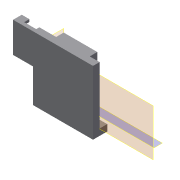
# Autodesk Inventor part: 10_Minispim_Base
Saved by Autodesk Inventor 2019 (Build 230136000, 136)
## iProperties
Created: 2019-08-27
Part Number: 10_Minispim_Base
Material: Generic
Document SubType Name: Modeling
Designer: diederichbenedict
Density: 1 g/cm^3
Appearance: Default
Author: diederichbenedict
Autodesk Inventor part; units mm, degrees
ref_plane "YZ Plane" through (0, 0, 0) normal (1, 0, 0) x (0, 1, 0)
ref_plane "XZ Plane" through (0, 0, 0) normal (0, 1, 0) x (-1, 0, 0)
ref_plane "XY Plane" through (0, 0, 0) normal (0, 0, 1) x (1, 0, 0)
ref_plane "Work Plane1" through (0, 0, 0) normal (0, 0, 1) x (1, 0, 0)
sketch "Sketch1" plane through (0, 0, 0) normal (0, 0, 1) x (1, 0, 0)
  line L0 (73, -36.65) -> (-73, -36.65) construction
  line L1 (73, 36.65) -> (73, -36.65) construction
  line L2 (-73, 36.65) -> (73, 36.65) construction
  line L3 (-73, -36.65) -> (-73, 36.65) construction
  line L4 (-66.8632, 12.8749) -> (-66.8632, 14.232) construction
  line L5 (-66.8632, 14.232) -> (-61.4969, 10.9795) construction
  line L6 (-61.4969, 10.9795) -> (-57.2382, 10.9795) construction
  line L7 (-57.2382, 10.9795) -> (-57.2382, 9.7003) construction
  line L8 (-57.2382, 9.7003) -> (-61.3643, 9.7003) construction
  line L9 (-61.3643, 9.7003) -> (-66.8632, 6.4478) construction
  line L10 (-66.8632, 6.4478) -> (-66.8632, 7.8674) construction
  line L11 (-66.8632, 7.8674) -> (-62.6279, 10.3477) construction
  line L12 (-62.6279, 10.3477) -> (-66.8632, 12.8749) construction
  spline S0 degree 2 poles (-57.9402, -12.888) (-57.519, -13.3482) (-57.0666, -14.5182) (-57.0666, -15.3995) knots 0 0 0 1 2 2 2 construction
  spline S1 degree 2 poles (-57.0666, -15.3995) (-57.0666, -16.4447) (-57.5034, -17.9111) (-57.8154, -18.5585) knots 0 0 0 1 2 2 2 construction
  line L13 (-57.8154, -18.5585) -> (-59.4221, -18.5585) construction
  line L14 (-59.4221, -18.5585) -> (-59.4221, -18.4649) construction
  spline S2 degree 2 poles (-59.4221, -18.4649) (-58.8294, -17.8331) (-58.1742, -16.2341) (-58.1742, -15.4931) knots 0 0 0 1 2 2 2 construction
  spline S3 degree 2 poles (-58.1742, -15.4931) (-58.1742, -14.4324) (-59.0555, -13.3482) (-59.7809, -13.3482) knots 0 0 0 1 2 2 2 construction
  spline S4 degree 2 poles (-59.7809, -13.3482) (-60.3581, -13.3482) (-61.0757, -13.9176) (-61.2551, -14.5338) knots 0 0 0 1 2 2 2 construction
  spline S5 degree 2 poles (-61.2551, -14.5338) (-61.3799, -14.9784) (-61.5515, -15.7193) (-61.6919, -16.2731) knots 0 0 0 1 2 2 2 construction
  spline S6 degree 2 poles (-61.6919, -16.2731) (-61.8245, -16.7723) (-62.2223, -17.5601) (-62.5421, -17.8643) knots 0 0 0 1 2 2 2 construction
  spline S7 degree 2 poles (-62.5421, -17.8643) (-62.8619, -18.1607) (-63.7199, -18.4883) (-64.2814, -18.4883) knots 0 0 0 1 2 2 2 construction
  spline S8 degree 2 poles (-64.2814, -18.4883) (-65.4514, -18.4883) (-67.0348, -16.6631) (-67.0348, -15.2514) knots 0 0 0 1 2 2 2 construction
  spline S9 degree 2 poles (-67.0348, -15.2514) (-67.0348, -14.4402) (-66.715, -13.005) (-66.4108, -12.3888) knots 0 0 0 1 2 2 2 construction
  line L15 (-66.4108, -12.3888) -> (-64.882, -12.3888) construction
  line L16 (-64.882, -12.3888) -> (-64.882, -12.4824) construction
  spline S10 degree 2 poles (-64.882, -12.4824) (-65.3032, -12.9426) (-65.9272, -14.3778) (-65.9272, -15.1656) knots 0 0 0 1 2 2 2 construction
  spline S11 degree 2 poles (-65.9272, -15.1656) (-65.9272, -16.0547) (-65.0926, -17.1545) (-64.414, -17.1545) knots 0 0 0 1 2 2 2 construction
  spline S12 degree 2 poles (-64.414, -17.1545) (-63.8057, -17.1545) (-63.0803, -16.5071) (-62.9165, -15.8987) knots 0 0 0 1 2 2 2 construction
  spline S13 degree 2 poles (-62.9165, -15.8987) (-62.8073, -15.4931) (-62.5265, -14.3154) (-62.4095, -13.9254) knots 0 0 0 1 2 2 2 construction
  spline S14 degree 2 poles (-62.4095, -13.9254) (-62.1053, -12.9348) (-60.8807, -12.0144) (-59.9837, -12.0144) knots 0 0 0 1 2 2 2 construction
  spline S15 degree 2 poles (-59.9837, -12.0144) (-59.4143, -12.0144) (-58.3224, -12.4746) (-57.9402, -12.888) knots 0 0 0 1 2 2 2 construction
  spline S16 degree 2 poles (-67.066, -7.0069) (-67.066, -6.0241) (-66.3796, -4.4486) (-65.7634, -3.9026) knots 0 0 0 1 2 2 2 construction
  spline S17 degree 2 poles (-65.7634, -3.9026) (-65.1238, -3.3566) (-63.2519, -2.7482) (-62.0507, -2.7482) knots 0 0 0 1 2 2 2 construction
  spline S18 degree 2 poles (-62.0507, -2.7482) (-60.8807, -2.7482) (-58.9854, -3.341) (-58.3458, -3.9026) knots 0 0 0 1 2 2 2 construction
  spline S19 degree 2 poles (-58.3458, -3.9026) (-57.675, -4.4954) (-57.0354, -6.0631) (-57.0354, -7.0069) knots 0 0 0 1 2 2 2 construction
  spline S20 degree 2 poles (-57.0354, -7.0069) (-57.0354, -7.9819) (-57.6984, -9.5419) (-58.3458, -10.1113) knots 0 0 0 1 2 2 2 construction
  spline S21 degree 2 poles (-58.3458, -10.1113) (-58.9854, -10.665) (-60.8651, -11.2578) (-62.0507, -11.2578) knots 0 0 0 1 2 2 2 construction
  spline S22 degree 2 poles (-62.0507, -11.2578) (-63.2597, -11.2578) (-65.1004, -10.6572) (-65.7634, -10.1035) knots 0 0 0 1 2 2 2 construction
  spline S23 degree 2 poles (-65.7634, -10.1035) (-66.403, -9.5419) (-67.066, -7.9741) (-67.066, -7.0069) knots 0 0 0 1 2 2 2 construction
  line L17 (-66.8632, 5.543) -> (-57.2382, 5.543) construction
  line L18 (-57.2382, 5.543) -> (-57.2382, 4.1078) construction
  line L19 (-57.2382, 4.1078) -> (-65.5372, -0.1509) construction
  line L20 (-65.5372, -0.1509) -> (-57.2382, -0.1509) construction
  line L21 (-57.2382, -0.1509) -> (-57.2382, -1.3442) construction
  line L22 (-57.2382, -1.3442) -> (-66.8632, -1.3442) construction
  line L23 (-66.8632, -1.3442) -> (-66.8632, 0.4731) construction
  line L24 (-66.8632, 0.4731) -> (-59.2427, 4.3496) construction
  line L25 (-59.2427, 4.3496) -> (-66.8632, 4.3496) construction
  line L26 (-66.8632, 4.3496) -> (-66.8632, 5.543) construction
  line L27 (-75, -25.3081) -> (-75, -38.65) construction
  line L28 (-75, -38.65) -> (75, -38.65) construction
  line L29 (-75, 38.65) -> (-75, -16.9919) construction
  line L30 (75, 38.65) -> (-75, 38.65) construction
  line L31 (-151.75, -50.65) -> (-11.75, -50.65)
  line L32 (-11.75, -50.65) -> (-11.75, 59.35)
  line L33 (-11.75, 59.35) -> (-151.75, 59.35)
  line L34 (-151.75, 59.35) -> (-151.75, -50.65)
  line L35 (-146.75, 47.05) -> (-146.75, 14.683) construction
  line L36 (-11.75, -50.65) -> (-75, -50.65)
  line L37 (-75, -50.65) -> (-75, 59.35)
  line L38 (-75, 59.35) -> (-11.75, 59.35)
  line L39 (-11.75, 59.35) -> (-11.75, -50.65)
  point P0 (0, 0)
  dimension "d0" = 140
  dimension "d1" = 110
  dimension "d2" = 12
  dimension "d3" = 5
  constraints: 16 end point, 4 parallel, 2 horizontal, 2 perpendicular, 1 point on line
  measures "d0" distance of L33.end L32.end
  measures "d1" distance of L32.end L31.end
  measures "d2" distance between parallel lines of L31 L28
  measures "d3" distance between parallel lines of L35 L34
ref_plane "Work Plane2" through (-137.8164, 12.7477, 6.4) normal (0, 0, 1) x (1, 0, 0)
extrude "Extrusion1" add sketch "Sketch1" along normal up to surface (6.4 mm away) contours L37 L33 L32 L31
sketch "Sketch2" plane through (0, 0, 0) normal (0, 0, -1) x (-1, 0, 0)
  line L0 (11.75, -50.65) -> (11.75, 59.35) projected
  line L1 (75, -50.65) -> (11.75, -50.65) projected
  line L2 (75, 59.35) -> (75, -50.65) projected
  line L3 (11.75, 59.35) -> (75, 59.35) projected
  line L4 (75, 38.65) -> (-75, 38.65) projected
  line L5 (75, -38.65) -> (-75, -38.65) projected
  line L6 (75, 59.35) -> (75, -50.65) projected
  line L7 (75, 59.35) -> (28.75, 59.35)
  line L8 (28.75, 59.35) -> (28.75, 39.65)
  line L9 (28.75, 39.65) -> (75, 39.65)
  line L10 (75, 39.65) -> (75, 59.35)
  line L11 (75, -50.65) -> (11.75, -50.65) projected
  line L12 (11.75, -50.65) -> (11.75, 59.35) projected
  line L13 (75, -50.65) -> (11.75, -50.65)
  line L14 (11.75, -50.65) -> (11.75, -39.65)
  line L15 (11.75, -39.65) -> (75, -39.65)
  line L16 (75, -39.65) -> (75, -50.65)
  point P0 (0, 0)
  dimension "d6" = 1
  dimension "d7" = 1
  dimension "d8" = 17
  constraints: 16 end point, 4 parallel, 2 horizontal, 2 perpendicular, 1 point on line
  measures "d6" distance between parallel lines of L9 L4
  measures "d7" distance between parallel lines of L15 L5
  measures "d8" distance between parallel lines of L0 L8
ref_plane "Work Plane3" through (-75.3762, -41.3829, -13.1) normal (0, 0, -1) x (0, 1, 0)
extrude "Extrusion2" add sketch "Sketch2" along normal up to surface (13.1 mm away) contours L0 L15 L2 L1 | L3 L2 L9 L8
sketch "Sketch3" plane through (-75, 59.35, 6.4) normal (0, 1, 0) x (1, 0, 0)
  arc A0 (-14.75, 0) -> (-4.75, 10) centre (-14.75, 10) ccw projected
  arc A1 (-71.75, 10) -> (-61.75, 0) centre (-61.75, 10) ccw projected
  line L0 (-71.75, 10) -> (-74.3413, 10)
  line L1 (-74.3413, 10) -> (-74.3413, 0)
  line L2 (-74.3413, 0) -> (-61.75, 0)
  line L3 (-14.75, 0) -> (0, 0)
  line L4 (0, 0) -> (0, 6.4)
  line L5 (0, 19.5) -> (0, 0) projected
  line L6 (-5.4205, 6.4) -> (0, 6.4)
  point P0 (75, 6.4)
  constraints: 12 end point, 3 perpendicular, 2 point on line, 1 horizontal, 1 point on circle
ref_plane "Work Plane4" through (-135.51, 6.95, -15.2395) normal (0, -1, 0) x (1, 0, 0)
extrude "Extrusion3" add sketch "Sketch3" against normal up to surface (52.4 mm away)
sketch "Sketch4" plane through (-75, -50.65, 6.4) normal (0, 0, 1) x (1, 0, 0)
  line L0 (-74.3413, 57.6) -> (-61.75, 57.6) projected
  line L1 (-61.75, 110) -> (-61.75, 57.6) projected
  line L2 (-61.75, 110) -> (-74.3413, 110) projected
  line L3 (-74.3413, 110) -> (-74.3413, 57.6) projected
  line L4 (63.25, 0) -> (0, 0) projected
  line L5 (63.25, 110) -> (63.25, 0) projected
  line L6 (63.25, 110) -> (-14.75, 110) projected
  line L7 (-14.75, 110) -> (-14.75, 57.6) projected
  line L8 (-14.75, 57.6) -> (0, 57.6) projected
  line L9 (0, 0) -> (0, 57.6) projected
  line L10 (-61.75, 110) -> (-61.75, 57.6) projected
  line L11 (-14.75, 57.6) -> (0, 57.6) projected
  line L12 (-61.75, 110) -> (-14.75, 110)
  line L13 (-14.75, 110) -> (-14.75, 57.6)
  line L14 (-14.75, 57.6) -> (-61.75, 57.6)
  line L15 (-61.75, 57.6) -> (-61.75, 110)
  line L16 (0, 57.6) -> (-40, 57.6)
  line L17 (-40, 57.6) -> (-40, 0)
  line L18 (-40, 0) -> (0, 0)
  line L19 (0, 0) -> (0, 57.6)
  point P0 (75, 50.65)
  dimension "d13" = 40
  constraints: 16 end point, 4 parallel, 2 horizontal, 2 perpendicular
  measures "d13" distance of L18.end L17.end
extrude "Extrusion4" add sketch "Sketch4" along normal blind 5
ref_plane "Work Plane5" through (-139.1935, 55.05, -12.427) normal (0, 1, 0) x (0, 0, 1)
sketch "Sketch5" plane through (-28.75, 59.35, 0) normal (0, 1, 0) x (1, 0, 0)
  line L0 (-61, -6.4) -> (-46.25, -6.4) projected
  line L1 (17, 0) -> (17, -11.4) projected
  line L2 (17, 0) -> (0, 0) projected
  line L3 (0, 0) -> (0, 13.1) projected
  line L4 (0, 13.1) -> (-46.25, 13.1) projected
  line L5 (-46.25, 13.1) -> (-46.25, 0) projected
  line L6 (-51.6705, 0) -> (-46.25, 0) projected
  arc A0 (-61, -6.4) -> (-51.6705, 0) centre (-61, 3.6) ccw projected
  line L7 (-61, -6.4) -> (-108, -6.4) projected
  arc A1 (-118, 3.6) -> (-108, -6.4) centre (-108, 3.6) ccw projected
  line L8 (-120.5913, 3.6) -> (-118, 3.6) projected
  line L9 (-120.5913, 3.6) -> (-120.5913, -11.4) projected
  line L10 (17, -11.4) -> (-120.5913, -11.4) projected
  line L11 (-46.25, 13.1) -> (-57.8775, 13.1)
  line L12 (-57.8775, 13.1) -> (-57.8775, 0)
  line L13 (-57.8775, 0) -> (-86.7528, 0)
  line L14 (-86.7528, 0) -> (-86.7528, -5.376)
  line L15 (-86.7528, -5.376) -> (-107.463, -5.376)
  line L16 (-107.463, -5.376) -> (-107.463, 3.6)
  line L17 (-107.463, 3.6) -> (-118, 3.6)
  point P0 (28.75, 0)
  constraints: 14 end point, 6 perpendicular, 1 horizontal
extrude "Extrusion5" add sketch "Sketch5" against normal up to surface (4.3 mm away) contours L5 L6 A0 L7 A1 L17 L16 L15 L14 L13 L12 L11
sketch "Sketch6" plane through (-75, -50.65, 6.4) normal (0, 0, -1) x (-1, 0, 0)
  line L0 (61.75, 105.7) -> (14.75, 105.7) projected
  line L1 (14.75, 105.7) -> (14.75, 57.6) projected
  line L2 (14.75, 57.6) -> (0, 57.6) projected
  line L3 (0, 0) -> (0, 57.6) projected
  line L4 (40, 0) -> (0, 0) projected
  line L5 (40, 57.6) -> (40, 0) projected
  line L6 (61.75, 57.6) -> (40, 57.6) projected
  line L7 (61.75, 105.7) -> (61.75, 57.6) projected
  line L8 (40, 57.6) -> (40, 0) projected
  line L9 (40, 47.989) -> (0, 47.989)
  line L10 (0, 47.989) -> (0, 42.989)
  line L11 (0, 42.989) -> (40, 42.989)
  line L12 (40, 42.989) -> (40, 47.989)
  line L13 (40, 0) -> (0, 0) projected
  line L14 (0, 42.989) -> (5, 42.989)
  line L15 (5, 42.989) -> (5, 0)
  line L16 (5, 0) -> (0, 0)
  line L17 (0, 0) -> (0, 42.989)
  point P0 (-75, 50.65)
  dimension "d18" = 5
  dimension "d19" = 5
  constraints: 16 end point, 4 parallel, 3 point on line, 2 horizontal, 2 perpendicular
  measures "d18" distance of L10.end L9.end
  measures "d19" distance of L15.end L16.end
extrude "Extrusion6" add sketch "Sketch6" along normal up to surface (19.5 mm away) contours L5 L11 L3 L9 | L11 L15 L4 L3
ref_plane "Work Plane6" through (-94.75, 13.95, -5.6) normal (1, 0, 0) x (0, -1, 0)
sketch "Sketch7" plane through (-94.75, 13.95, -5.6) normal (1, 0, 0) x (0, -1, 0)
  line L0 (14.7, 6) -> (30.1, 6)
  line L1 (14.7, -6) -> (30.1, -6)
  line L2 (12.1377, -0.0565) -> (37.0671, -0.0565)
  line L3 (14.7, -0.0565) -> (22.7, -0.0565)
  line L4 (22.7, -0.0565) -> (22.7, 6.2435)
  line L5 (22.7, 6.2435) -> (14.7, 6.2435)
  line L6 (14.7, 6.2435) -> (14.7, -0.0565)
  line L7 (21.611, -12) -> (21.611, 7.5) projected
  line L8 (21.611, -0.0565) -> (20.1319, -0.0565)
  line L9 (20.1319, -0.0565) -> (20.1319, 6.8333)
  line L10 (20.1319, 6.8333) -> (21.611, 6.8333)
  line L11 (21.611, 6.8333) -> (21.611, -0.0565)
  point P0 (13.95, -5.6)
  dimension "d22" = 8
  dimension "d23" = 6.3
  constraints: 22 end point, 5 horizontal, 4 parallel, 3 point on line, 2 perpendicular, 4 other
  measures "d22" distance of L5.end L4.end
  measures "d23" distance of L4.end L3.end
revolve "Revolution1" cut sketch "Sketch7" angle 360 about axis through (-94.75, 1.8123, -5.5435) along (0, -1, 0)
ref_plane "Work Plane7" through (-61.9, -21.15, -5.6) normal (0, -1, 0) x (1, 0, 0)
sketch "Sketch8" plane through (-61.9, -21.15, -5.6) normal (0, -1, 0) x (1, 0, 0)
  line L0 (-15.1, -6.34) -> (-15.1, 6.34) construction
  line L1 (-16.3, -6.34) -> (-15.1, -6.34) construction
  arc A0 (-18.2, 0) -> (-16.3, -6.34) centre (-3.4124, 0.9769) ccw construction
  arc A1 (-16.3, 6.34) -> (-18.2, 0) centre (-3.4124, -0.9769) ccw construction
  line L2 (-16.3, 6.34) -> (-15.1, 6.34) construction
  line L3 (-18.1, 12) -> (-18.1, -7.5) construction
  line L4 (-13.1, 5.6) -> (-13.1, -7.5) construction
  line L5 (-18.1, -5.7052) -> (-13.1, -5.7052) construction
  line L6 (-13.1, -5.7052) -> (-13.1, 5.6) construction
  line L7 (-13.1, 5.6) -> (-18.1, 5.6) construction
  line L8 (-18.1, 5.6) -> (-18.1, -5.7052) construction
  line L9 (-22.253, 0) -> (-12.4028, 0) construction
  line L10 (-16.4447, -6.59) -> (-14.85, -6.59)
  line L11 (-14.85, -6.59) -> (-14.85, 6.59)
  line L12 (-14.85, 6.59) -> (-16.4447, 6.59)
  arc A2 (-16.4447, 6.59) -> (-18.4505, 0) centre (-3.4124, -0.9769) ccw
  arc A3 (-18.4505, 0) -> (-16.4447, -6.59) centre (-3.4124, 0.9769) ccw
  line L13 (-14.85, -5.7052) -> (-13.1, -5.7052)
  line L14 (-18.5205, 5.6) -> (-13.1, 5.6) projected
  line L15 (-14.85, 5.6) -> (-13.1, 5.6)
  line L16 (-14.85, 0) -> (-13.1, 0)
  line L17 (-13.1, 0) -> (-13.1, -5.4209)
  line L18 (-13.1, -5.4209) -> (-14.85, -5.4209)
  line L19 (-14.85, -5.4209) -> (-14.85, 0)
  line L20 (-14.85, 0) -> (-18.4505, 0)
  line L21 (-16.4447, -6.59) -> (-18.1, -6.7731)
  line L22 (-18.1, -6.7731) -> (-18.1, -2.3957)
  point P0 (61.9, 5.6)
  dimension "d25" = 0.25
  constraints: 38 end point, 9 point on circle, 9 point on line, 5 horizontal, 4 centre point, 4 parallel, 3 collinear, 2 perpendicular, 1 midpoint, 11 other
  measures "d25" radial gap between concentric circles of A0 A3
revolve "Revolution2" cut sketch "Sketch8" angle 360 about axis through (-76.75, -21.15, -5.6) along (-1, 0, 0) contours A3 L20 L11 L10 | L21 L22 A3 | L11 L16 L17 L18
body "Solid1"
